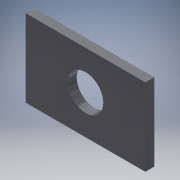
# Autodesk Inventor part: 20-028Z1
Saved by Autodesk Inventor 2018 (Build 220105000, 105)
## iProperties
Shininess: 64.0
Length Units: 11269
Angle Units: 11279
Time Units: 11290
Mass Units: 11286
Length Display Precision: 3
Angle Display Precision: 2
Compacted: True
Created: 2003-01-07
Part Number: 20-028Z1
Material: Steel, High Strength Low Alloy
Vendor: PARKER IPS
Document SubType Name: Modeling
Designer: Autodesk, Inc.
Description: FLAT PLATE FASTENER (w/o screw)
Catalog Web Link: http://www.parker.com/ead/cm1.asp?cmid=809
Mass: 6.62064 g
Surface Area: 10.7273 cm^2
Volume: 0.844469 cm^3
Density: 7.84 g/cm^3
Appearance: Metal-Steel (Polished)
Density: 0.0
Volumn: 0.0
Area: 0.0
PropertySet Name: Model Information
Control State: 0
Master: False
Checked Out: False
CAGE: 08JJ3
NEXT HIGHER ASSY 01: ---
Author: Autodesk, Inc.
Autodesk Inventor part; units mm, degrees
ref_plane "YZ Plane" through (0, 0, 0) normal (1, 0, 0) x (0, 1, 0)
ref_plane "XZ Plane" through (0, 0, 0) normal (0, 1, 0) x (-1, 0, 0)
ref_plane "XY Plane" through (0, 0, 0) normal (0, 0, 1) x (1, 0, 0)
sketch "Sketch1" plane through (0, 0, 0) normal (0, 0, 1) x (1, 0, 0)
  line L0 (-13.5, -8.75) -> (13.5, -8.75)
  line L1 (13.5, -8.75) -> (13.5, 8.75)
  line L2 (13.5, 8.75) -> (-13.5, 8.75)
  line L3 (-13.5, 8.75) -> (-13.5, -8.75)
  line L4 (0, 0) -> (0, 8.75) construction
  line L5 (0, 0) -> (13.5, 0) construction
  circle A0 centre (0, 0) radius 4
  dimension "d0" = 27
  dimension "d2" = 8
  dimension "d3" = 17.5
  constraints: 12 end point, 3 perpendicular, 2 midpoint, 2 parallel, 1 centre point, 1 coincident, 1 horizontal, 1 other
  measures "d0" distance of L0.start L0.end
  measures "d2" diameter of A0
  measures "d3" distance of L0.end L1.end
extrude "Extrusion1" add sketch "Sketch1" along normal mid plane 2
body "Solid1"
